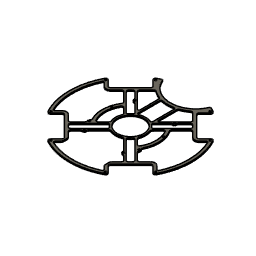
Frame_upperside v15 (Autodesk Fusion 360 design; units mm, degrees)
Autodesk Fusion 360 part; units mm, degrees
(part 1 of 2)
sketch "スケッチ1" plane through (0, 0, 0) normal (0, 0, 1) x (1, 0, 0)
  circle A0 centre (0, 0) radius 108
  circle A1 centre (0, 115.48) radius 45
  line L0 (0, 0) -> (76.3675, 76.3675)
  line L1 (0, 0) -> (108, 0) construction
  line L2 (0, 0) -> (76.3675, -76.3675)
  line L3 (76.3675, 76.3675) -> (58.5484, 58.5484)
  line L4 (76.3675, 76.3675) -> (96.1665, 56.5685)
  line L5 (76.3675, 76.3675) -> (56.5685, 96.1665)
  line L6 (96.1665, 56.5685) -> (78.3474, 38.7495)
  line L7 (78.3474, 38.7495) -> (58.5484, 58.5484)
  line L8 (56.5685, 96.1665) -> (38.7495, 78.3474)
  line L9 (38.7495, 78.3474) -> (58.5484, 58.5484)
  line L10 (56.5685, -96.1665) -> (38.7495, -78.3474)
  line L11 (38.7495, -78.3474) -> (58.5484, -58.5484)
  line L12 (78.3474, -38.7495) -> (58.5484, -58.5484)
  line L13 (96.1665, -56.5685) -> (78.3474, -38.7495)
  line L14 (76.3675, -76.3675) -> (96.1665, -56.5685)
  line L15 (76.3675, -76.3675) -> (56.5685, -96.1665)
  line L16 (0, 2.5) -> (0, 20)
  line L17 (-56.5685, -96.1665) -> (-38.7495, -78.3474)
  line L18 (-38.7495, -78.3474) -> (-58.5484, -58.5484)
  line L19 (-78.3474, -38.7495) -> (-58.5484, -58.5484)
  line L20 (-96.1665, -56.5685) -> (-78.3474, -38.7495)
  line L21 (-76.3675, -76.3675) -> (-96.1665, -56.5685)
  line L22 (-76.3675, -76.3675) -> (-56.5685, -96.1665)
  line L23 (0, 0) -> (-76.3675, -76.3675)
  line L24 (0, 0) -> (-76.3675, 76.3675)
  line L25 (-38.7495, 78.3474) -> (-58.5484, 58.5484)
  line L26 (-78.3474, 38.7495) -> (-58.5484, 58.5484)
  line L27 (-56.5685, 96.1665) -> (-38.7495, 78.3474)
  line L28 (-76.3675, 76.3675) -> (-56.5685, 96.1665)
  line L29 (-76.3675, 76.3675) -> (-96.1665, 56.5685)
  line L30 (-96.1665, 56.5685) -> (-78.3474, 38.7495)
  line L31 (-96.1665, 56.5685) -> (-99.7021, 53.033)
  line L32 (-99.7021, 53.033) -> (-78.3474, 31.6784)
  line L33 (-78.3474, 31.6784) -> (-31.6784, 78.3474)
  line L34 (-31.6784, 78.3474) -> (-53.033, 99.7021)
  line L35 (-53.033, 99.7021) -> (-56.5685, 96.1665)
  line L36 (-99.7021, -53.033) -> (-78.3474, -31.6784)
  line L37 (-78.3474, -31.6784) -> (-31.6784, -78.3474)
  line L38 (-31.6784, -78.3474) -> (-53.033, -99.7021)
  line L39 (-96.1665, -56.5685) -> (-99.7021, -53.033)
  line L40 (-53.033, -99.7021) -> (-56.5685, -96.1665)
  line L41 (96.1665, -56.5685) -> (99.7021, -53.033)
  line L42 (99.7021, -53.033) -> (78.3474, -31.6784)
  line L43 (78.3474, -31.6784) -> (31.6784, -78.3474)
  line L44 (31.6784, -78.3474) -> (53.033, -99.7021)
  line L45 (53.033, -99.7021) -> (56.5685, -96.1665)
  line L46 (96.1665, 56.5685) -> (99.7021, 53.033)
  line L47 (99.7021, 53.033) -> (78.3474, 31.6784)
  line L48 (78.3474, 31.6784) -> (31.6784, 78.3474)
  line L49 (31.6784, 78.3474) -> (53.033, 99.7021)
  line L50 (53.033, 99.7021) -> (56.5685, 96.1665)
  circle A2 centre (0, 0) radius 103
  line L51 (0, 115.48) -> (0, 70.48)
  line L52 (-31.6784, -78.3474) -> (-32.739, -77.2868)
  circle A3 centre (-48.1818, -92.7295) radius 1.65
  line L53 (-78.3474, -31.6784) -> (-77.2868, -32.739)
  circle A4 centre (-92.7295, -48.1818) radius 1.65
  line L54 (31.6784, -78.3474) -> (32.739, -77.2868)
  line L55 (32.739, -77.2868) -> (54.0937, -98.6414)
  circle A5 centre (48.1818, -92.7295) radius 1.65
  line L56 (78.3474, -31.6784) -> (77.2868, -32.739)
  line L57 (77.2868, -32.739) -> (98.6414, -54.0937)
  circle A6 centre (92.7295, -48.1818) radius 1.65
  line L58 (-99.7021, 53.033) -> (-98.6414, 54.0937)
  circle A7 centre (-92.7295, 48.1818) radius 1.65
  circle A8 centre (92.7295, -48.1818) radius 1.65
  circle A9 centre (48.1818, 92.7295) radius 1.65
  circle A10 centre (-92.7295, 48.1818) radius 1.65
  line L59 (31.6784, 78.3474) -> (32.739, 77.2868)
  circle A11 centre (48.1818, -92.7295) radius 1.65
  circle A12 centre (92.7295, 48.1818) radius 1.65
  circle A13 centre (-48.1818, 92.7295) radius 1.65
  line L60 (-31.6784, 78.3474) -> (-28.9756, 81.0502)
  line L61 (38.7495, 78.3474) -> (38.0423, 77.6403)
  line L62 (-38.7495, 78.3474) -> (-38.0423, 77.6403)
  line L63 (-38.0423, 77.6403) -> (-40.4063, 75.2764)
  line L64 (38.0423, 77.6403) -> (40.4063, 75.2764)
  line L65 (0, 70.48) -> (0, 65.48)
  circle A14 centre (0, 115.48) radius 50
  line L66 (0, 65.48) -> (0, 42.88)
  line L67 (0, 42.88) -> (-35, 42.88)
  line L68 (0, 42.88) -> (35, 42.88)
  line L69 (35, 42.88) -> (-35, 42.88)
  line L70 (-35, 42.88) -> (-35, -47.12)
  line L71 (-35, -47.12) -> (35, -47.12)
  line L72 (35, -47.12) -> (35, 42.88)
  line L73 (-55.0129, -55.0129) -> (-51.1238, -58.902)
  line L74 (-51.1238, -58.902) -> (62.4375, 54.6594)
  line L75 (-51.1238, -58.902) -> (-49.0025, -61.0233)
  line L76 (-49.0025, -61.0233) -> (64.5588, 52.538)
  line L77 (-35, 42.88) -> (35, 42.88)
  line L78 (35, 42.88) -> (35, -42.12)
  line L79 (35, -42.12) -> (-35, -42.12)
  line L80 (-35, -42.12) -> (-35, 42.88)
  line L81 (-58.902, -51.1238) -> (54.6594, 62.4375)
  line L82 (-61.0233, -49.0025) -> (52.538, 64.5588)
  line L83 (-58.5484, 58.5484) -> (-54.6594, 62.4375)
  line L84 (-54.6594, 62.4375) -> (62.4375, -54.6594)
  line L85 (-54.6594, 62.4375) -> (-52.538, 64.5588)
  line L86 (-52.538, 64.5588) -> (64.5588, -52.538)
  line L87 (-64.5588, 52.538) -> (52.538, -64.5588)
  line L88 (-62.4375, 54.6594) -> (54.6594, -62.4375)
  circle A15 centre (-35, 42.88) radius 2.5
  circle A16 centre (-35, 42.88) radius 1.65
  circle A17 centre (35, 42.88) radius 1.65
  circle A18 centre (35, 42.88) radius 2.5
  circle A19 centre (0, 0) radius 50
  line L89 (-50, 0) -> (-45, 0)
  circle A20 centre (0, 0) radius 45
  circle A21 centre (-47.5, 0) radius 1.65
  circle A22 centre (47.5, 0) radius 1.65
  circle A23 centre (0, 0) radius 26.5
  line L90 (-26.5, 0) -> (-23.5, 0)
  circle A24 centre (0, 0) radius 23.5
  circle A25 centre (-25, 0) radius 2.5
  circle A26 centre (-25, 0) radius 1.65
  circle A27 centre (25, 0) radius 2.5
  circle A28 centre (25, 0) radius 1.65
  line L91 (0, 67.98) -> (-6, 67.98)
  line L92 (-6, 67.98) -> (-6, 25.8118)
  line L93 (-6, 67.98) -> (-9, 67.98)
  line L94 (-9, 67.98) -> (-9, 24.9249)
  line L95 (0, 67.98) -> (6, 67.98)
  line L96 (6, 67.98) -> (6, 25.8118)
  line L97 (6, 67.98) -> (9, 67.98)
  line L98 (9, 67.98) -> (9, 24.9249)
  line L99 (-38.7495, -78.3474) -> (-31.6784, -78.3474)
  line L100 (-35.2139, -78.3474) -> (-38.7495, -78.3474)
  line L101 (-36.9817, -78.3474) -> (-35.2139, -78.3474)
  line L102 (-36.9817, -78.3474) -> (-36.9817, -73.0441)
  line L103 (-36.9817, -73.0441) -> (-36.9817, -83.6507)
  line L104 (-36.9817, -78.3474) -> (-38.7495, -78.3474)
  line L105 (-37.8656, -78.3474) -> (-37.8656, -72.1602)
  line L106 (-37.8656, -78.3474) -> (-37.8656, -84.5346)
  line L107 (37.8656, -78.3474) -> (37.8656, -72.1602)
  line L108 (36.9817, -73.0441) -> (36.9817, -83.6507)
  line L109 (37.8656, -78.3474) -> (37.8656, -84.5346)
  circle A29 centre (35, -47.12) radius 1.65
  circle A30 centre (35, -47.12) radius 2.5
  circle A31 centre (-35, -47.12) radius 1.65
  circle A32 centre (-35, -47.12) radius 2.5
  line L110 (47.5, 0) -> (35, 0)
  line L111 (37.2574, 25.2366) -> (37.2574, 0)
  line L112 (37.2574, 12.6183) -> (48.3816, 12.6183)
  line L113 (43.1947, 12.6183) -> (48.3816, 12.6183)
  circle A33 centre (45.7881, 12.6183) radius 1.65
  circle A34 centre (-45.7881, 12.6183) radius 1.65
  line L114 (37.2574, -25.2366) -> (43.1638, -25.2366)
  circle A35 centre (40.2106, -25.2366) radius 1.65
  circle A36 centre (-40.2106, -25.2366) radius 1.65
  line L115 (-45.7881, 12.6183) -> (-45.7881, -33.7673)
  line L116 (-40.2106, -25.2366) -> (-45.7881, -25.2366)
  circle A37 centre (-45.7881, -25.2366) radius 1.65
  circle A38 centre (-45.7881, -25.2366) radius 2.5
  circle A39 centre (-45.7881, -22.7366) radius 2.5
  circle A40 centre (-45.7881, -22.7366) radius 1.65
  circle A41 centre (45.7881, -22.7366) radius 2.5
  circle A42 centre (45.7881, -22.7366) radius 1.65
  line L117 (-45.7881, -33.7673) -> (-45.7881, -38.01)
  line L118 (-45.7881, -38.01) -> (-45.7881, -33.7673)
  circle A43 centre (-45.7881, -35.8886) radius 2.5
  circle A44 centre (-45.7881, -35.8886) radius 1.65
  circle A45 centre (45.7881, -35.8886) radius 2.5
  circle A46 centre (45.7881, -35.8886) radius 1.65
  dimension "d1" = 216
  dimension "d2" = 90
  dimension "d4" = 45
  dimension "d5" = 25.2
  dimension "d6" = 28
  dimension "d7" = 28
  dimension "d9" = 25.2
  dimension "d10" = 28
  dimension "d11" = 25.2
  dimension "d12" = 28
  dimension "d13" = 5
  dimension "d14" = 30.2
  dimension "d15" = 66
  dimension "d16" = 30.2
  dimension "d40" = 1.5
  dimension "d42" = 3.3
  dimension "d43" = 1.5
  dimension "d45" = 3.3
  dimension "d46" = 1.5
  dimension "d48" = 3.3
  dimension "d49" = 1.5
  dimension "d51" = 3.3
  dimension "d52" = 1.5
  dimension "d54" = 3.3
  dimension "d57" = 1.5
  dimension "d77" = 1
  dimension "d173" = 5
  dimension "d174" = 22.6
  dimension "d175" = 35
  dimension "d176" = 35
  dimension "d177" = 90
  dimension "d178" = 5.5
  dimension "d179" = 3
  dimension "d180" = 85
  dimension "d183" = 5.5
  dimension "d184" = 3
  dimension "d185" = 5
  dimension "d186" = 3.3
  dimension "d187" = 3.3
  dimension "d188" = 5
  dimension "d189" = 100
  dimension "d190" = 5
  dimension "d191" = 3.3
  dimension "d192" = 3.3
  dimension "d193" = 53
  dimension "d194" = 3
  dimension "d195" = 5
  dimension "d196" = 3.3
  dimension "d197" = 6
  dimension "d198" = 3
  dimension "d199" = 6
  dimension "d200" = 3
  dimension "d205" = 3.3
  dimension "d206" = 5
  dimension "d207" = 3.3
  dimension "d208" = 5
  dimension "d209" = 90
  dimension "d210" = 3.3
  dimension "d211" = 3.3
  dimension "d236" = 3.3
  dimension "d237" = 5
  dimension "d238" = 3.3
  dimension "d239" = 5
  dimension "d240" = 3.3
  constraint coincident A0.centre L0.start
  constraint horizontal L1
  constraint coincident A0 L0.end
  constraint coincident A0 L2.end
  constraint perpendicular L0 L2
  constraint perpendicular L2 L3
  constraint perpendicular L3 L4
  constraint perpendicular L0 L5
  constraint perpendicular L4 L6
  constraint perpendicular L6 L7
  constraint perpendicular L5 L8
  constraint perpendicular L8 L9
  constraint symmetric L0.end L1 L2.end
  constraint symmetric L1 L4.end L13.start
  constraint symmetric L1 L5.end L10.start
  constraint symmetric L1 L6.end L12.start
  constraint symmetric L1 L3.end L11.end
  constraint symmetric L1 L8.end L10.end
  constraint symmetric A0.centre L16 L0.start
  constraint symmetric L0.end L16 L24.end
  constraint symmetric L2.end L16 L21.start
  constraint symmetric L4.end L16 L29.end
  constraint symmetric L5.end L16 L27.start
  constraint symmetric L6.end L16 L26.start
  constraint symmetric L3.end L16 L25.end
  constraint symmetric L8.end L16 L25.start
  constraint symmetric L10.start L16 L17.start
  constraint symmetric L10.end L16 L17.end
  constraint symmetric L11.end L16 L18.end
  constraint symmetric L12.start L16 L19.start
  constraint symmetric L13.start L16 L20.start
  constraint perpendicular L30 L31
  constraint perpendicular L26 L32
  constraint perpendicular L32 L33
  constraint perpendicular L33 L34
  constraint symmetric L1 L27.start L17.start
  constraint symmetric L1 L29.end L20.start
  constraint symmetric L1 L31.end L36.start
  constraint symmetric L1 L32.end L36.end
  constraint symmetric L1 L33.end L37.end
  constraint symmetric L1 L34.end L38.end
  constraint symmetric L16 L27.start L5.end
  constraint symmetric L16 L29.end L4.end
  constraint symmetric L16 L31.end L46.end
  constraint symmetric L16 L32.end L47.end
  constraint symmetric L16 L33.end L48.end
  constraint symmetric L16 L34.end L49.end
  constraint symmetric L16 L36.start L41.end
  constraint symmetric L16 L36.end L42.end
  constraint symmetric L16 L37.end L43.end
  constraint symmetric L16 L38.end L44.end
  constraint symmetric L16 L20.start L13.start
  constraint symmetric L16 L17.start L10.start
  constraint coincident A1.centre L51.start
  constraint coincident A1 L51.end
  constraint vertical L51
  constraint coincident L37 L52.end
  constraint perpendicular L36 L53
  constraint perpendicular L44 L54
  constraint coincident L45 L55.end
  constraint perpendicular L45 L55
  constraint perpendicular L42 L56
  constraint coincident L41 L57.end
  constraint perpendicular L41 L57
  constraint perpendicular L32 L58
  constraint perpendicular L49 L59
  constraint coincident A1 L60.end
  constraint perpendicular L34 L60
  constraint perpendicular L9 L61
  constraint perpendicular L25 L62
  constraint perpendicular L62 L63
  constraint perpendicular L63 L64
  constraint parallel L51 L65
  constraint concentric A1 A14
  constraint coincident L65.end A14
  constraint parallel L65 L66
  constraint perpendicular L65 L67
  constraint perpendicular L66 L68
  constraint horizontal L69
  constraint vertical L70
  constraint horizontal L71
  constraint vertical L72
  constraint midpoint L37 L73.start
  constraint perpendicular L23 L73
  constraint coincident L7 L74.end
  constraint perpendicular L7 L74
  constraint coincident L37 L75.end
  constraint coincident L7 L76.end
  constraint perpendicular L7 L76
  constraint horizontal L77
  constraint vertical L78
  constraint horizontal L79
  constraint vertical L80
  constraint symmetric L23 L73.end L81.start
  constraint symmetric L23 L74.end L81.end
  constraint symmetric L23 L75.end L82.start
  constraint symmetric L23 L76.end L82.end
  constraint coincident L12 L84.end
  constraint perpendicular L12 L84
  constraint perpendicular L84 L85
  constraint coincident L12 L86.end
  constraint perpendicular L12 L86
  constraint symmetric L2 L83.end L88.start
  constraint symmetric L2 L84.end L88.end
  constraint symmetric L2 L85.end L87.start
  constraint symmetric L2 L86.end L87.end
  constraint coincident L67.end L69.end
  constraint concentric A15 A16
  constraint coincident L68.end L69.start
  constraint concentric A17 A18
  constraint concentric A0 A19
  constraint coincident A19 L89.start
  constraint horizontal L89
  constraint concentric A19 A20
  constraint coincident L89.end A20
  constraint midpoint L89 A21.centre
  constraint coincident L1 A22.centre
  constraint coincident A23 L90.start
  constraint horizontal L90
  constraint coincident L90.end A24
  constraint midpoint L90 A25.centre
  constraint concentric A25 A26
  constraint symmetric L16 A25 A27
  constraint symmetric L16 A26 A28
  constraint midpoint L65 L91.start
  constraint perpendicular L65 L91
  constraint coincident A23 L92.end
  constraint perpendicular L67 L92
  constraint perpendicular L92 L93
  constraint coincident A23 L94.end
  constraint perpendicular L93 L94
  constraint perpendicular L65 L95
  constraint coincident A23 L96.end
  constraint perpendicular L77 L96
  constraint perpendicular L96 L97
  constraint coincident A23 L98.end
  constraint perpendicular L97 L98
  constraint midpoint L99 L100.start
  constraint midpoint L100 L101.start
  constraint coincident L37 L102.end
  constraint perpendicular L101 L102
  constraint coincident L38 L103.end
  constraint perpendicular L99 L103
  constraint midpoint L104 L105.start
  constraint coincident L37 L105.end
  constraint perpendicular L100 L105
  constraint coincident L38 L106.end
  constraint perpendicular L100 L106
  constraint symmetric L16 L102.end L108.start
  constraint symmetric L16 L103.end L108.end
  constraint symmetric L16 L105.start L107.start
  constraint symmetric L16 L105.end L107.end
  constraint symmetric L16 L106.end L109.end
  constraint coincident L71.end L72.start
  constraint concentric A29 A30
  constraint coincident L70.end L71.start
  constraint concentric A31 A32
  constraint coincident A22.centre L110.start
  constraint coincident L72 L110.end
  constraint coincident L1 L110.end
  constraint coincident L78 L110.end
  constraint coincident A20 L111.start
  constraint coincident L76 L111.start
  constraint coincident L1 L111.end
  constraint midpoint L111 L112.start
  constraint coincident A19 L112.end
  constraint perpendicular L111 L112
  constraint coincident L112 L113.start
  constraint coincident A20 L113.start
  constraint midpoint L113 A33.centre
  constraint symmetric L16 A33 A34
  constraint coincident A20 L114.start
  constraint coincident L86 L114.start
  constraint coincident A19 L114.end
  constraint horizontal L114
  constraint midpoint L114 A35.centre
  constraint symmetric L16 A35 A36
  constraint coincident A34.centre L115.start
  constraint coincident L82 L115.end
  constraint vertical L115
  constraint coincident A36.centre L116.start
  constraint coincident L115 L116.end
  constraint perpendicular L115 L116
  constraint coincident L116.end A37.centre
  constraint concentric A37 A38
  constraint coincident L115 A39.centre
  constraint coincident A38 A39.centre
  constraint coincident L116.end A39
  constraint concentric A39 A40
  constraint symmetric L16 A39 A41
  constraint symmetric L16 A40 A42
  constraint coincident L81 L117.end
  constraint parallel L115 L117
  constraint midpoint L117 A43.centre
  constraint concentric A43 A44
  constraint symmetric L16 A43 A45
  constraint symmetric L16 A44 A46
  measures "d1" diameter of A0
  measures "d2" diameter of A1
  measures "d4" angle of L0 L1
  measures "d5" distance of L0.end L3.end
  measures "d6" distance of L0.end L4.end
  measures "d7" distance of L0.end L5.end
  measures "d9" distance of L4.end L6.end
  measures "d10" distance of L6.end L3.end
  measures "d11" distance of L5.end L8.end
  measures "d12" distance of L8.end L3.end
  measures "d13" distance of L29.end L31.end
  measures "d14" distance of L31.end L32.end
  measures "d15" distance of L32.end L33.end
  measures "d16" distance of L33.end L34.end
  measures "d40" distance of L37.end L52.end
  measures "d42" diameter of A3
  measures "d43" distance of L36.end L53.end
  measures "d45" diameter of A4
  measures "d46" distance of L43.end L54.end
  measures "d48" diameter of A5
  measures "d49" distance of L42.end L56.end
  measures "d51" diameter of A6
  measures "d52" distance of L31.end L58.end
  measures "d54" diameter of A7
  measures "d57" distance of L48.end L59.end
  measures "d77" distance of L8.end L61.end
  measures "d173" distance of L51.end L65.end
  measures "d174" distance of L65.end L66.end
  measures "d175" distance of L66.end L67.end
  measures "d176" distance of L66.end L68.end
  measures "d177" distance of L68.end L71.end
  measures "d178" distance of L73.start L73.end
  measures "d179" distance of L73.end L75.end
  measures "d180" distance of L67.end L79.end
  measures "d183" distance of L25.end L83.end
  measures "d184" distance of L83.end L85.end
  measures "d185" diameter of A15
  measures "d186" diameter of A16
  measures "d187" diameter of A17
  measures "d188" diameter of A18
  measures "d189" diameter of A19
  measures "d190" distance of L89.start L89.end
  measures "d191" diameter of A21
  measures "d192" diameter of A22
  measures "d193" diameter of A23
  measures "d194" distance of L90.start L90.end
  measures "d195" diameter of A25
  measures "d196" diameter of A26
  measures "d197" distance of L91.start L91.end
  measures "d198" distance of L91.end L93.end
  measures "d199" distance of L91.start L95.end
  measures "d200" distance of L95.end L97.end
  measures "d205" diameter of A29
  measures "d206" diameter of A30
  measures "d207" diameter of A31
  measures "d208" diameter of A32
  measures "d209" angle of L110 L111
  measures "d210" diameter of A33
  measures "d211" diameter of A35
  measures "d236" diameter of A37
  measures "d237" diameter of A38
  measures "d238" diameter of A40
  measures "d239" diameter of A43
  measures "d240" diameter of A44
extrude "押し出し7" add sketch "スケッチ1" along normal blind 2 contours A0 L42 L47 A2 A6 A8 A12 | A0 L6 L47 A2 A12 | A0 L42 L57 A6 A8 | A0 L13 A2 L57 A6 A8 | L6 L7 L47 L48 A2 A12 L76 | L47 A2 A12 | L42 A2 A6 A8 | A0 L8 L49 A2 A9 | L12 L13 L43 A2 L57 A6 A8 L86 | L42 L43 A2 L56 L57 A6 A8 | A0 L49 A2 A9 A14 | L8 L9 L48 L49 A2 A9 L59 A14 L82 | L0 L7 L48 L74 | L0 L9 L48 L81 | L7 L48 L74 L76 | A0 L10 A2 L55 A5 A11 | A0 A1 A2 A14 | L9 L48 L81 L82 | L48 L74 L76 A19 | A0 L44 L55 A5 A11 | L10 L11 L43 A2 L55 A5 A11 L87 L107 L109 | L2 L11 L43 L88 | L2 L12 L43 L84 | L12 L43 L84 L86 | A1 L48 L49 A2 L59 L65 A14 L95 L97 L98 | L49 A2 A14 | L49 A2 A9 | L48 L68 L69 L77 L81 L82 A18 | L76 A19 A20 L112 L113 A33 | L74 L76 A19 A20 | A0 L38 L44 A2 A3 A5 A11 | L11 L43 L87 L88 | L43 L84 L86 A45 | L48 L49 L59 A14 | A0 L34 A2 A13 A14 | A0 A1 A2 A14 | L72 L78 L81 A17 A18 | L68 L69 L77 L81 A17 A18 | L72 L74 L76 L78 A20 | A19 A20 L112 L113 A33 L114 A35 A41 | A0 L17 L38 A2 A3 | L44 A2 L55 A5 A11 L109 | L43 L72 L87 L88 A30 | L84 L86 A45 A46 | A1 L33 L60 L65 A14 L91 L93 L94 | A0 L27 L34 A2 A13 | L34 A2 A14 | A1 L34 A2 L60 A14 | L68 L69 L77 L81 L82 A18 A19 | L72 L78 L81 A17 A18 | L81 L82 A19 A20 | L68 L69 L77 L81 A17 A18 | L72 L74 L76 L78 A23 | L44 A2 A5 A11 | L44 L55 L108 L109 | L43 L55 L107 L108 L109 | L84 L86 A19 A45 | L84 L86 A19 A20 | L72 L79 L87 L88 A30 | L84 L86 A46 | L65 A14 L95 L96 | L65 A14 L91 L92 | A14 A19 L96 L98 | A14 L96 L97 L98 | L34 A2 A13 | L25 L27 L33 L34 A2 A13 A14 L86 | L33 L34 A14 | L0 L74 A23 A24 | L0 L81 A23 A24 | L81 L82 A20 A23 | L76 A23 A24 A27 | L74 L76 A23 A24 | A19 A41 A42 | L17 L38 A2 A3 L99 L100 L104 L106 | L38 A2 A3 | L71 L87 A29 A30 | L72 L87 A29 A30 | L87 L88 A19 A20 | L79 L87 L88 A19 | L72 L78 L84 L86 A20 | L84 L86 A45 A46 | L86 A19 L114 A35 | L72 L87 A29 A30 | A14 L92 L93 L94 | A19 A20 L96 L98 | L81 L82 A23 A24 | L72 L78 L84 L86 A23 | A23 A24 A27 A28 | A19 A42 | A0 L20 L36 A2 A4 | L18 L23 L37 L73 L75 L99 L100 L104 L105 | L71 L87 A29 A30 | L2 L88 A23 A24 | L2 L84 A23 A24 | L87 L88 A20 A23 | A14 A19 L92 L94 | L68 L69 L77 A20 L96 L98 | A0 L30 L32 A2 A7 A10 | L33 L67 L69 L77 L84 L86 A15 | L25 L33 L84 L85 L86 | L68 L69 L77 A23 L96 L98 | L82 L86 A23 A24 | L84 L86 A23 A24 | L86 A23 A24 A27 | A23 A24 A28 | A0 L32 L36 A2 A4 A7 A10 | L19 L20 L23 L36 L37 A2 L53 A4 | L37 L99 L100 L102 L103 L104 L105 | L38 L99 L100 L103 L104 L106 | L87 L88 A23 A24 | A19 A20 L92 L94 | L26 L30 L32 L33 A2 A7 A10 L87 | L24 L25 L33 L83 L84 | L24 L26 L33 L88 | L67 L69 L77 L84 L86 A15 A19 | A23 A24 A27 A28 | L76 L87 A23 A24 | L67 L69 L77 A20 L92 L94 | L26 L33 L87 L88 | L67 L69 L77 L84 A15 A16 | L70 L80 L84 A15 A16 | L67 L69 L77 L84 A15 A16 | L84 L86 A19 A20 | L84 L86 A23 A24 | L36 A2 A4 | L37 L81 L82 A43 | L37 L70 L74 L75 L76 A32 | L71 L76 A31 A32 | L71 L76 A31 A32 | L74 L76 A23 A24 | L74 L76 A20 A23 | L67 L69 L77 A23 L92 L94 | L32 A2 A7 A10 | L33 L87 L88 A19 | L70 L80 L84 A15 A16 | L84 L86 A20 A23 | L24 L84 A23 A24 | L81 L82 A19 A20 | L81 L82 A19 A43 | L81 L82 L117 L118 A43 A44 | L70 L74 L76 L79 A32 | L70 L76 A31 A32 | L70 L76 A31 A32 | L74 L76 L79 A19 | L74 L76 A19 A20 | L23 L74 A23 A24 | L87 L88 A19 A20 | L24 L88 A23 A24 | L81 L82 L117 L118 A43 A44 | L70 L80 L81 L82 A20 | L82 A19 L89 A20 L115 A38 A39 | L81 L117 L118 A44 | L23 L81 A23 A24 | L87 A19 L89 A20 A21 | L70 L80 L87 L88 A20 | L87 L88 A23 A24 | L70 L80 L81 L82 A23 | L81 L117 L118 A44 | L82 L117 L118 A44 | L81 L82 A23 A24 | A19 L89 A21 L115 | L70 L80 L87 L88 A23 | L87 A23 A24 A25 | L82 L117 L118 A44 | A19 A38 A39 | L82 A23 A24 A25 | A23 A24 A25 A26 | A19 A38 A39 A40 | A19 A38 A39 A40 | A23 A24 A25 A26 | A23 L90 A24 A26 | A19 A38 A40 | A19 A38 A40 | A23 L90 A24 A26 picked at (92.3485, 46.0877) picked at (46.0877, 92.3485) picked at (-46.0859, 92.3935) picked at (43.8614, -23.2917) picked at (-46.0859, -92.3935) picked at (44.6077, -22.1956) picked at (-92.3485, -46.0877) picked at (-92.3485, 46.0877)
fillet "フィレット21" radius 3 16 edges at (-93.5553, 53.9574, 1) (-53.9574, 93.5553, 1) (-38.7495, 78.3474, 1) (-78.3474, 38.7495, 1) (-93.5553, -53.9574, 1) (-78.3474, -38.7495, 1) (-38.7495, -78.3474, 1) (-53.9574, -93.5553, 1) (53.9574, -93.5553, 1) (93.5553, -53.9574, 1) (78.3474, -38.7495, 1) (38.7495, -78.3474, 1) (78.3474, 38.7495, 1) (93.5553, 53.9574, 1) (38.7495, 78.3474, 1) (53.9574, 93.5553, 1)
fillet "フィレット22" radius 2 6 edges at (-92.3273, 45.6582, 1) (-92.3273, -45.6582, 1) (-45.6582, -92.3273, 1) (45.6582, -92.3273, 1) (92.3273, -45.6582, 1) (92.3273, 45.6582, 1)
fillet "フィレット23" radius 8 4 edges at (-78.3474, 31.6784, 1) (-78.3474, -31.6784, 1) (78.3474, -31.6784, 1) (78.3474, 31.6784, 1)
fillet "フィレット24" radius 5 4 edges at (-36.9817, -83.6507, 1) (-36.9817, -73.0441, 1) (36.9817, -83.6507, 1) (36.9817, -73.0441, 1)
fillet "フィレット25" radius 3 16 edges at (-58.902, -51.1238, 1) (-61.0233, -49.0025, 1) (-51.1238, -58.902, 1) (-49.0025, -61.0233, 1) (49.0025, -61.0233, 1) (51.1238, -58.902, 1) (58.902, -51.1238, 1) (61.0233, -49.0025, 1) (-61.0233, 49.0025, 1) (-58.902, 51.1238, 1) (-51.1238, 58.902, 1) (-49.0025, 61.0233, 1) (61.0233, 49.0025, 1) (58.902, 51.1238, 1) (51.1238, 58.902, 1) (49.0025, 61.0233, 1)
fillet "フィレット27" radius 3 4 edges at (-40.8511, -28.8303, 1) (-37.2574, -25.2366, 1) (-40.8511, 28.8303, 1) (-37.2574, 25.2366, 1)
fillet "フィレット27" radius 3 4 edges at (37.2574, -25.2366, 1) (40.8511, -28.8303, 1) (37.2574, 25.2366, 1) (40.8511, 28.8303, 1)
fillet "フィレット28" radius 5 8 edges at (-36.8167, -48.8375, 1) (-33.2825, -45.3033, 1) (33.2825, -45.3033, 1) (36.8167, -48.8375, 1) (-33.2839, 41.0621, 1) (-36.8179, 44.5961, 1) (33.2839, 41.0621, 1) (36.8179, 44.5961, 1)
fillet "フィレット29" radius 3 2 edges at (-32.5229, 77.5029, 1) (32.5229, 77.5029, 1)
fillet "フィレット30" radius 1.5 2 edges at (-42.0574, 99.4745, 1) (42.0574, 99.4745, 1)
fillet "フィレット33" radius 5 2 edges at (23.7586, -11.7378, 1) (23.7586, 11.7378, 1)
fillet "フィレット33" radius 3 1 edges at (11.7378, -23.7586, 1)
sketch "スケッチ5" plane through (0, 0, 2) normal (0, 0, 1) x (-1, 0, 0)
  arc A0 (-43.4817, -98.8602) -> (-41.4947, -98.0676) centre (-42.8778, -97.4871) ccw
  arc A1 (41.4947, -98.0676) -> (-41.4947, -98.0676) centre (0, -115.48) ccw
  arc A2 (41.4947, -98.0676) -> (43.4817, -98.8602) centre (42.8778, -97.4871) ccw
  arc A3 (43.4817, -98.8602) -> (50.4167, -95.51) centre (0, 0) ccw
  arc A4 (50.4167, -95.51) -> (51.1376, -90.7356) centre (49.0163, -92.8569) ccw
  line L0 (51.1376, -90.7356) -> (40.8708, -80.4688)
  arc A5 (40.8708, -76.2261) -> (40.8708, -80.4688) centre (42.9921, -78.3474) ccw
  line L1 (40.8708, -76.2261) -> (76.2261, -40.8708)
  arc A6 (80.4688, -40.8708) -> (76.2261, -40.8708) centre (78.3474, -42.9921) ccw
  line L2 (80.4688, -40.8708) -> (90.7356, -51.1376)
  arc A7 (90.7356, -51.1376) -> (95.51, -50.4167) centre (92.8569, -49.0163) ccw
  arc A8 (95.51, -50.4167) -> (95.51, 50.4167) centre (0, 0) ccw
  arc A9 (95.51, 50.4167) -> (90.7356, 51.1376) centre (92.8569, 49.0163) ccw
  line L3 (90.7356, 51.1376) -> (80.4688, 40.8708)
  arc A10 (76.2261, 40.8708) -> (80.4688, 40.8708) centre (78.3474, 42.9921) ccw
  line L4 (76.2261, 40.8708) -> (40.8708, 76.2261)
  arc A11 (40.8708, 80.4688) -> (40.8708, 76.2261) centre (42.9921, 78.3474) ccw
  line L5 (40.8708, 80.4688) -> (51.1376, 90.7356)
  arc A12 (51.1376, 90.7356) -> (50.4167, 95.51) centre (49.0163, 92.8569) ccw
  arc A13 (50.4167, 95.51) -> (-50.4167, 95.51) centre (0, 0) ccw
  arc A14 (-50.4167, 95.51) -> (-51.1376, 90.7356) centre (-49.0163, 92.8569) ccw
  line L6 (-51.1376, 90.7356) -> (-40.8708, 80.4688)
  arc A15 (-40.8708, 76.2261) -> (-40.8708, 80.4688) centre (-42.9921, 78.3474) ccw
  line L7 (-40.8708, 76.2261) -> (-76.2261, 40.8708)
  arc A16 (-80.4688, 40.8708) -> (-76.2261, 40.8708) centre (-78.3474, 42.9921) ccw
  line L8 (-80.4688, 40.8708) -> (-90.7356, 51.1376)
  arc A17 (-90.7356, 51.1376) -> (-95.51, 50.4167) centre (-92.8569, 49.0163) ccw
  arc A18 (-95.51, 50.4167) -> (-95.51, -50.4167) centre (0, 0) ccw
  arc A19 (-95.51, -50.4167) -> (-90.7356, -51.1376) centre (-92.8569, -49.0163) ccw
  line L9 (-90.7356, -51.1376) -> (-80.4688, -40.8708)
  arc A20 (-76.2261, -40.8708) -> (-80.4688, -40.8708) centre (-78.3474, -42.9921) ccw
  line L10 (-76.2261, -40.8708) -> (-40.8708, -76.2261)
  arc A21 (-40.8708, -80.4688) -> (-40.8708, -76.2261) centre (-42.9921, -78.3474) ccw
  line L11 (-40.8708, -80.4688) -> (-51.1376, -90.7356)
  arc A22 (-51.1376, -90.7356) -> (-50.4167, -95.51) centre (-49.0163, -92.8569) ccw
  arc A23 (-50.4167, -95.51) -> (-43.4817, -98.8602) centre (0, 0) ccw
  arc A24 (-38.4462, 71.5797) -> (-36.9817, 75.1152) centre (-41.9817, 75.1152) ccw
  line L12 (-36.9817, 75.1152) -> (-36.9817, 81.5797)
  arc A25 (-36.9817, 81.5797) -> (-38.4462, 85.1152) centre (-41.9817, 81.5797) ccw
  line L13 (-38.4462, 85.1152) -> (-43.658, 90.3271)
  arc A26 (-43.0803, 93.5579) -> (-43.658, 90.3271) centre (-42.2438, 91.7413) ccw
  arc A27 (43.0803, 93.5579) -> (-43.0803, 93.5579) centre (0, 0) ccw
  arc A28 (43.658, 90.3271) -> (43.0803, 93.5579) centre (42.2438, 91.7413) ccw
  line L14 (43.658, 90.3271) -> (38.4462, 85.1152)
  arc A29 (38.4462, 85.1152) -> (36.9817, 81.5797) centre (41.9817, 81.5797) ccw
  line L15 (36.9817, 81.5797) -> (36.9817, 75.1152)
  arc A30 (36.9817, 75.1152) -> (38.4462, 71.5797) centre (41.9817, 75.1152) ccw
  line L16 (38.4462, 71.5797) -> (46.8812, 63.1446)
  arc A31 (46.8812, 58.902) -> (46.8812, 63.1446) centre (44.7599, 61.0233) ccw
  line L17 (46.8812, 58.902) -> (39.0462, 51.0671)
  arc A32 (35.1702, 49.6142) -> (39.0462, 51.0671) centre (35.5107, 54.6026) ccw
  arc A33 (35.1702, 49.6142) -> (32.5058, 46.9498) centre (35, 47.12) ccw
  arc A34 (31.0529, 43.0738) -> (32.5058, 46.9498) centre (27.5174, 46.6093) ccw
  line L18 (31.0529, 43.0738) -> (11.7378, 23.7586)
  arc A35 (11.7378, 23.7586) -> (-9.9511, 24.5606) centre (0, 0) ccw
  arc A36 (-13.199, 25.2198) -> (-9.9511, 24.5606) centre (-11.0776, 27.3411) ccw
  line L19 (-13.199, 25.2198) -> (-31.0529, 43.0738)
  arc A37 (-32.5058, 46.9498) -> (-31.0529, 43.0738) centre (-27.5174, 46.6093) ccw
  arc A38 (-32.5058, 46.9498) -> (-35.1702, 49.6142) centre (-35, 47.12) ccw
  arc A39 (-39.0462, 51.0671) -> (-35.1702, 49.6142) centre (-35.5107, 54.6026) ccw
  line L20 (-39.0462, 51.0671) -> (-46.8812, 58.902)
  arc A40 (-46.8812, 63.1446) -> (-46.8812, 58.902) centre (-44.7599, 61.0233) ccw
  line L21 (-46.8812, 63.1446) -> (-38.4462, 71.5797)
  arc A41 (-72.6906, -37.3352) -> (-84.0043, -37.3352) centre (-78.3474, -42.9921) ccw
  line L22 (-84.0043, -37.3352) -> (-90.3271, -43.658)
  arc A42 (-93.5579, -43.0803) -> (-90.3271, -43.658) centre (-91.7413, -42.2438) ccw
  arc A43 (-93.5579, 43.0803) -> (-93.5579, -43.0803) centre (0, 0) ccw
  arc A44 (-90.3271, 43.658) -> (-93.5579, 43.0803) centre (-91.7413, 42.2438) ccw
  line L23 (-90.3271, 43.658) -> (-84.0043, 37.3352)
  arc A45 (-84.0043, 37.3352) -> (-72.6906, 37.3352) centre (-78.3474, 42.9921) ccw
  line L24 (-72.6906, 37.3352) -> (-63.1446, 46.8812)
  arc A46 (-58.902, 46.8812) -> (-63.1446, 46.8812) centre (-61.0233, 44.7599) ccw
  line L25 (-58.902, 46.8812) -> (-42.5942, 30.5734)
  arc A47 (-42.1845, 26.8416) -> (-42.5942, 30.5734) centre (-44.7155, 28.4521) ccw
  arc A48 (-42.1845, 26.8416) -> (-42.1845, -26.8416) centre (0, 0) ccw
  arc A49 (-42.5942, -30.5734) -> (-42.1845, -26.8416) centre (-44.7155, -28.4521) ccw
  line L26 (-42.5942, -30.5734) -> (-58.902, -46.8812)
  arc A50 (-63.1446, -46.8812) -> (-58.902, -46.8812) centre (-61.0233, -44.7599) ccw
  line L27 (-63.1446, -46.8812) -> (-72.6906, -37.3352)
  arc A51 (72.6906, 37.3352) -> (84.0043, 37.3352) centre (78.3474, 42.9921) ccw
  line L28 (84.0043, 37.3352) -> (90.3271, 43.658)
  arc A52 (93.5579, 43.0803) -> (90.3271, 43.658) centre (91.7413, 42.2438) ccw
  arc A53 (93.5579, -43.0803) -> (93.5579, 43.0803) centre (0, 0) ccw
  arc A54 (90.3271, -43.658) -> (93.5579, -43.0803) centre (91.7413, -42.2438) ccw
  line L29 (90.3271, -43.658) -> (84.0043, -37.3352)
  arc A55 (84.0043, -37.3352) -> (72.6906, -37.3352) centre (78.3474, -42.9921) ccw
  line L30 (72.6906, -37.3352) -> (63.1446, -46.8812)
  arc A56 (58.902, -46.8812) -> (63.1446, -46.8812) centre (61.0233, -44.7599) ccw
  line L31 (58.902, -46.8812) -> (42.5942, -30.5734)
  arc A57 (42.1845, -26.8416) -> (42.5942, -30.5734) centre (44.7155, -28.4521) ccw
  arc A58 (42.1845, -26.8416) -> (42.1845, 26.8416) centre (0, 0) ccw
  arc A59 (42.5942, 30.5734) -> (42.1845, 26.8416) centre (44.7155, 28.4521) ccw
  line L32 (42.5942, 30.5734) -> (58.902, 46.8812)
  arc A60 (63.1446, 46.8812) -> (58.902, 46.8812) centre (61.0233, 44.7599) ccw
  line L33 (63.1446, 46.8812) -> (72.6906, 37.3352)
  line L34 (-22.2194, 14.4412) -> (-56.7807, 49.0025)
  arc A61 (-56.7807, 53.2451) -> (-56.7807, 49.0025) centre (-54.6594, 51.1238) ccw
  line L35 (-56.7807, 53.2451) -> (-53.2451, 56.7807)
  arc A62 (-49.0025, 56.7807) -> (-53.2451, 56.7807) centre (-51.1238, 54.6594) ccw
  line L36 (-49.0025, 56.7807) -> (-14.4412, 22.2194)
  arc A63 (-14.4412, 22.2194) -> (-22.2194, 14.4412) centre (0, 0) ccw
  circle A64 centre (-92.7295, 48.1818) radius 1.65
  circle A65 centre (-92.7295, -48.1818) radius 1.65
  circle A66 centre (-40.2106, 25.2366) radius 1.65
  line L37 (-34.5739, 22.5531) -> (-26.135, 14.1142)
  arc A67 (-24.9609, 8.8995) -> (-26.135, 14.1142) centre (-29.6706, 10.5787) ccw
  arc A68 (-24.9609, 8.8995) -> (-24.9609, -8.8995) centre (0, 0) ccw
  arc A69 (-26.135, -14.1142) -> (-24.9609, -8.8995) centre (-29.6706, -10.5787) ccw
  line L38 (-26.135, -14.1142) -> (-34.5739, -22.5531)
  arc A70 (-39.3163, -21.8912) -> (-34.5739, -22.5531) centre (-36.6953, -20.4318) ccw
  arc A71 (-39.3163, 21.8912) -> (-39.3163, -21.8912) centre (0, 0) ccw
  arc A72 (-34.5739, 22.5531) -> (-39.3163, 21.8912) centre (-36.6953, 20.4318) ccw
  circle A73 centre (-47.5, 0) radius 1.65
  line L39 (-56.7807, -49.0025) -> (-22.2194, -14.4412)
  arc A74 (-22.2194, -14.4412) -> (-14.4412, -22.2194) centre (0, 0) ccw
  line L40 (-14.4412, -22.2194) -> (-31.1442, -38.9224)
  arc A75 (-34.8932, -40.3823) -> (-31.1442, -38.9224) centre (-34.6797, -35.3868) ccw
  arc A76 (-34.8932, -40.3823) -> (-37.4977, -42.9868) centre (-35, -42.88) ccw
  arc A77 (-38.9576, -46.7358) -> (-37.4977, -42.9868) centre (-42.4932, -43.2003) ccw
  line L41 (-38.9576, -46.7358) -> (-49.0025, -56.7807)
  arc A78 (-53.2451, -56.7807) -> (-49.0025, -56.7807) centre (-51.1238, -54.6594) ccw
  line L42 (-53.2451, -56.7807) -> (-56.7807, -53.2451)
  arc A79 (-56.7807, -49.0025) -> (-56.7807, -53.2451) centre (-54.6594, -51.1238) ccw
  circle A80 centre (-48.1818, -92.7295) radius 1.65
  circle A81 centre (48.1818, -92.7295) radius 1.65
  arc A82 (23.7586, -11.7378) -> (23.7586, 11.7378) centre (0, 0) ccw
  line L43 (23.7586, 11.7378) -> (34.5739, 22.5531)
  arc A83 (39.3163, 21.8912) -> (34.5739, 22.5531) centre (36.6953, 20.4318) ccw
  arc A84 (39.3163, -21.8912) -> (39.3163, 21.8912) centre (0, 0) ccw
  arc A85 (34.5739, -22.5531) -> (39.3163, -21.8912) centre (36.6953, -20.4318) ccw
  line L44 (34.5739, -22.5531) -> (23.7586, -11.7378)
  circle A86 centre (48.1818, 92.7295) radius 1.65
  circle A87 centre (40.2106, 25.2366) radius 1.65
  circle A88 centre (35, 47.12) radius 1.65
  circle A89 centre (-35, 47.12) radius 1.65
  circle A90 centre (45.7881, -12.6183) radius 1.65
  circle A91 centre (35, -42.88) radius 1.65
  circle A92 centre (47.5, 0) radius 1.65
  line L45 (22.2194, -14.4412) -> (56.7807, -49.0025)
  arc A93 (56.7807, -53.2451) -> (56.7807, -49.0025) centre (54.6594, -51.1238) ccw
  line L46 (56.7807, -53.2451) -> (53.2451, -56.7807)
  arc A94 (49.0025, -56.7807) -> (53.2451, -56.7807) centre (51.1238, -54.6594) ccw
  line L47 (49.0025, -56.7807) -> (38.9576, -46.7358)
  arc A95 (37.4977, -42.9868) -> (38.9576, -46.7358) centre (42.4932, -43.2003) ccw
  arc A96 (37.4977, -42.9868) -> (34.8932, -40.3823) centre (35, -42.88) ccw
  arc A97 (31.1442, -38.9224) -> (34.8932, -40.3823) centre (34.6797, -35.3868) ccw
  line L48 (31.1442, -38.9224) -> (14.4412, -22.2194)
  arc A98 (14.4412, -22.2194) -> (22.2194, -14.4412) centre (0, 0) ccw
  circle A99 centre (92.7295, -48.1818) radius 1.65
  circle A100 centre (92.7295, 48.1818) radius 1.65
  line L49 (53.2451, 56.7807) -> (56.7807, 53.2451)
  arc A101 (56.7807, 49.0025) -> (56.7807, 53.2451) centre (54.6594, 51.1238) ccw
  line L50 (56.7807, 49.0025) -> (22.2194, 14.4412)
  arc A102 (22.2194, 14.4412) -> (14.4412, 22.2194) centre (0, 0) ccw
  line L51 (14.4412, 22.2194) -> (49.0025, 56.7807)
  arc A103 (53.2451, 56.7807) -> (49.0025, 56.7807) centre (51.1238, 54.6594) ccw
  line L52 (9, -66.2967) -> (9, -24.9249)
  line L53 (11.7378, -23.7586) -> (46.8812, -58.902)
  arc A104 (46.8812, -63.1446) -> (46.8812, -58.902) centre (44.7599, -61.0233) ccw
  line L54 (46.8812, -63.1446) -> (34.4346, -75.5912)
  arc A105 (30.4842, -75.8478) -> (34.4346, -75.5912) centre (32.3133, -73.4699) ccw
  arc A106 (30.4842, -75.8478) -> (9, -66.2967) centre (0, -115.48) ccw
  arc A107 (6, -65.8413) -> (-6, -65.8413) centre (0, -115.48) ccw
  line L55 (-6, -65.8413) -> (-6, -25.8118)
  arc A108 (-6, -25.8118) -> (6, -25.8118) centre (0, 0) ccw
  line L56 (6, -25.8118) -> (6, -65.8413)
  circle A109 centre (-45.7881, -12.6183) radius 1.65
  line L57 (-46.8812, -58.902) -> (-11.7378, -23.7586)
  line L58 (-9, -24.9249) -> (-9, -66.2967)
  arc A110 (-9, -66.2967) -> (-30.4842, -75.8478) centre (0, -115.48) ccw
  arc A111 (-34.4346, -75.5912) -> (-30.4842, -75.8478) centre (-32.3133, -73.4699) ccw
  line L59 (-34.4346, -75.5912) -> (-46.8812, -63.1446)
  arc A112 (-46.8812, -58.902) -> (-46.8812, -63.1446) centre (-44.7599, -61.0233) ccw
  circle A113 centre (-35, -42.88) radius 1.65
  circle A114 centre (0, 0) radius 23.5
  circle A115 centre (-48.1818, 92.7295) radius 1.65
  arc A116 (9, -24.9249) -> (11.7378, -23.7586) centre (0, 0) ccw
  arc A117 (-11.7378, -23.7586) -> (-9, -24.9249) centre (0, 0) ccw
extrude "押し出し8" add sketch "スケッチ5" against normal blind 2 contours A66 | A73 | A87 | A92